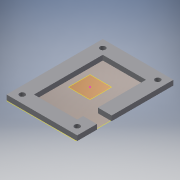
# Autodesk Inventor part: Pieza3
Saved by Autodesk Inventor 2017 (Build 210142000, 142)
## iProperties
Part Number: Pieza3
Material: Genérico
Document SubType Name: Modeling
Designer: user
Density: 1 g/cm^3
Appearance: Valor por defecto
Author: user
Autodesk Inventor part; units mm, degrees
ref_plane "YZ Plane" through (0, 0, 0) normal (1, 0, 0) x (0, 1, 0)
ref_plane "XZ Plane" through (0, 0, 0) normal (0, 1, 0) x (-1, 0, 0)
ref_plane "XY Plane" through (0, 0, 0) normal (0, 0, 1) x (1, 0, 0)
ref_plane "Plano de trabajo1" through (0, 0, 0) normal (0, 0, 1) x (1, 0, 0)
sketch "Boceto1" plane through (0, 0, 0) normal (0, 0, 1) x (1, 0, 0)
  line L0 (-22, -35) -> (22, -35) projected
  line L1 (-22, 35) -> (-22, -35) projected
  line L2 (22, 35) -> (-22, 35) projected
  line L3 (22, -35) -> (22, 35) projected
  line L4 (-36, -49) -> (36, -49) projected
  line L5 (36, -49) -> (36, 49) projected
  line L6 (36, 49) -> (-36, 49) projected
  line L7 (-36, 49) -> (-36, -49) projected
  line L8 (-36, -49) -> (36, -49)
  line L9 (36, -49) -> (36, 49)
  line L10 (36, 49) -> (-36, 49)
  line L11 (-36, 49) -> (-36, -49)
  line L12 (-22, -35) -> (22, -35)
  line L13 (22, 35) -> (-22, 35)
  line L14 (-22, 35) -> (-22, -35)
  circle A0 centre (28, -41) radius 2.75 projected
  circle A1 centre (-28, 41) radius 2.75 projected
  circle A2 centre (28, 41) radius 2.75 projected
  circle A3 centre (-28, -41) radius 2.75 projected
  line L15 (36, -49) -> (36, -29)
  line L16 (36, -29) -> (22, -29)
  line L17 (36, -29) -> (36, -14)
  line L18 (36, -14) -> (22, -14)
  line L19 (22, -35) -> (22, -29)
  line L20 (22, -14) -> (22, 35)
  point P0 (0, 0)
  dimension "d16" = 20
  dimension "d17" = 15
  dimension "d18" = 0
  constraints: 26 end point, 7 perpendicular, 5 parallel, 2 horizontal, 2 point on line
  measures "d16" distance of L8.end L15.end
  measures "d17" distance of L15.end L17.end
  measures "d18" distance between parallel lines of L3 L19
ref_plane "Plano de trabajo4" through (0, 0, 5) normal (0, 0, 1) x (1, 0, 0)
ref_plane "Plano de trabajo3" through (0, 0, 5) normal (0, 0, 1) x (1, 0, 0)
ref_plane "Plano de trabajo2" through (0, 0, 5) normal (0, 0, 1) x (1, 0, 0)
sketch "Boceto4" plane through (0, 0, 5) normal (0, 0, 1) x (1, 0, 0)
  point P0 (0, 0)
extrude "Extrusión2" add sketch "Boceto1" along normal blind 5 contours L0 L3 L16 L5 L4 L7 L6 L18 L2 L1
sketch "Boceto2" plane through (0, 0, 5) normal (0, 0, 1) x (1, 0, 0)
  point P0 (-28, 41)
  point P1 (28, 41)
  point P2 (28, -41)
  point P3 (-28, -41)
sketch "Boceto3" plane through (0, 0, 5) normal (0, 0, 1) x (1, 0, 0)
  point P0 (-28, 41)
  point P1 (28, 41)
  point P2 (28, -41)
  point P3 (-28, -41)
